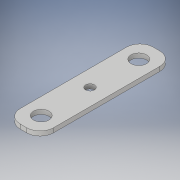
# Autodesk Inventor part: femur_v5
Saved by Autodesk Inventor 2019 (Build 230136000, 136)
## iProperties
Created: 2019-01-08
Part Number: femur_v5
Material: Generic
Document SubType Name: Modeling
Designer: Daniel
Density: 1 g/cm^3
Appearance: Default
Author: Daniel
Autodesk Inventor part; units mm, degrees
ref_plane "YZ Plane" through (0, 0, 0) normal (1, 0, 0) x (0, 1, 0)
ref_plane "XZ Plane" through (0, 0, 0) normal (0, 1, 0) x (-1, 0, 0)
ref_plane "XY Plane" through (0, 0, 0) normal (0, 0, 1) x (1, 0, 0)
sketch "Sketch1" plane through (0, 0, 0) normal (0, 1, 0) x (-1, 0, 0)
  line L0 (10.5, 0) -> (-10.5, 0) projected
  line L1 (0, -42) -> (0, 42) projected
  line L2 (7.5, -30) -> (-7.5, -30)
  line L3 (-7.5, -30) -> (-7.5, 30)
  line L4 (-7.5, 30) -> (7.5, 30)
  line L5 (7.5, 30) -> (7.5, -30)
  point P0 (0, 0)
  dimension "d0" = 15
  dimension "d1" = 60
  constraints: 8 end point, 2 parallel, 1 horizontal, 1 perpendicular, 2 other
  measures "d0" distance between parallel lines of L3 L5
  measures "d1" distance between parallel lines of L4 L2
extrude "Extrusion1" add sketch "Sketch1" along normal blind 2
fillet "Fillet1" radius 6 4 edges at (7.5, 1, -30) (-7.5, 1, -30) (-7.5, 1, 30) (7.5, 1, 30)
sketch "Sketch5" plane through (0, 2, 0) normal (0, 1, 0) x (1, 0, 0)
  arc A0 (1.5, -30) -> (7.5, -24) centre (1.5, -24) ccw projected
  line L0 (7.5, -24) -> (7.5, 24) projected
  arc A1 (7.5, 24) -> (1.5, 30) centre (1.5, 24) ccw projected
  line L1 (1.5, 30) -> (-1.5, 30) projected
  arc A2 (-1.5, 30) -> (-7.5, 24) centre (-1.5, 24) ccw projected
  line L2 (-7.5, 24) -> (-7.5, -24) projected
  arc A3 (-7.5, -24) -> (-1.5, -30) centre (-1.5, -24) ccw projected
  line L3 (-1.5, -30) -> (1.5, -30) projected
  point P0 (0, 0)
  point P1 (0, 0)
  constraints: 1 coincident
hole "Hole3" at (0, 2, 0) direction (0, -1, 0) diameter 4 end through all
sketch "Sketch6" plane through (0, 2, 0) normal (0, 1, 0) x (1, 0, 0)
  circle A0 centre (0, 0) radius 2 projected
  arc A1 (1.5, -30) -> (7.5, -24) centre (1.5, -24) ccw projected
  line L0 (7.5, -24) -> (7.5, 24) projected
  arc A2 (7.5, 24) -> (1.5, 30) centre (1.5, 24) ccw projected
  line L1 (1.5, 30) -> (-1.5, 30) projected
  arc A3 (-1.5, 30) -> (-7.5, 24) centre (-1.5, 24) ccw projected
  line L2 (-7.5, 24) -> (-7.5, -24) projected
  arc A4 (-7.5, -24) -> (-1.5, -30) centre (-1.5, -24) ccw projected
  line L3 (-1.5, -30) -> (1.5, -30) projected
  line L4 (0, 43.7397) -> (0, -43.7397) projected
  line L5 (-12.2397, 0) -> (12.2397, 0) projected
  point P0 (0, 22)
  point P1 (0, -22)
  dimension "d41" = 8
  dimension "d42" = 8
  constraints: 2 point on line
  measures "d41" distance from line of L1 point (0, 22)
  measures "d42" distance from line of L3 point (0, -22)
hole "Hole4" at (0, 2, -22) at (0, 2, 22) direction (0, -1, 0) diameter 7 end through all
body "Solid1"
